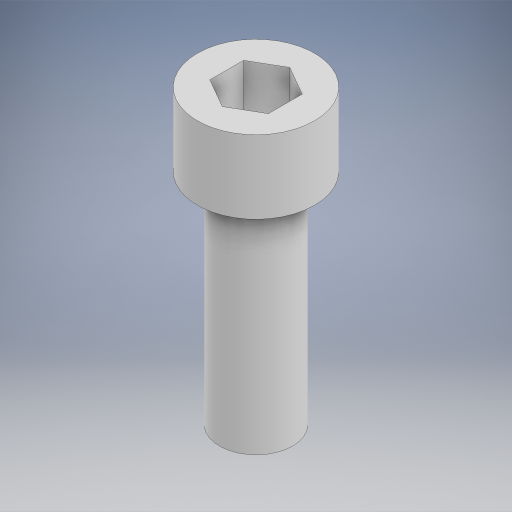
# Autodesk Inventor part: CE-2.1.5-01
Saved by Autodesk Inventor 2024 (Build 280153000, 153)
## iProperties
Created: 2024-01-31
Part Number: CE-2.1.5-01
Material: Generic
Document SubType Name: Modeling
Designer: Alex
Density: 1 g/cm^3
Appearance: Default
Author: Alex
Autodesk Inventor part; units mm, degrees
ref_plane "YZ Plane" through (0, 0, 0) normal (1, 0, 0) x (0, 1, 0)
ref_plane "XZ Plane" through (0, 0, 0) normal (0, 1, 0) x (-1, 0, 0)
ref_plane "XY Plane" through (0, 0, 0) normal (0, 0, 1) x (1, 0, 0)
sketch "Sketch1" plane through (0, 0, 0) normal (0, 0, 1) x (1, 0, 0)
  line L0 (0, 0) -> (0, 80)
  line L1 (0, 80) -> (16, 80)
  line L2 (16, 80) -> (16, 60)
  line L3 (16, 60) -> (10, 60)
  line L4 (10, 60) -> (10, 0)
  line L5 (0, 0) -> (10, 0)
  dimension "d" = 20
  dimension "HT" = 20
  dimension "Height" = 60
  dimension "HD" = 32
  constraints: 12 end point, 4 perpendicular, 1 horizontal, 1 vertical
  measures "d" diameter of L4 L0
  measures "HT" distance of L1.end L2.end
  measures "Height" distance of L3.end L4.end
  measures "HD" diameter of L2 L0
revolve "Revolution1" add sketch "Sketch1" angle 360 about axis through (0, 0, 0) along (0, 1, 0)
sketch "Sketch2" plane through (0, 80, 0) normal (0, 1, 0) x (1, 0, 0)
  line L0 (0, 9.2376) -> (8, 4.6188)
  line L1 (8, 4.6188) -> (8, -4.6188)
  line L2 (8, -4.6188) -> (0, -9.2376)
  line L3 (0, -9.2376) -> (-8, -4.6188)
  line L4 (-8, -4.6188) -> (-8, 4.6188)
  line L5 (-8, 4.6188) -> (0, 9.2376)
  point P0 (0, 0)
  point P1 (0, 0)
  dimension "HL" = 16
  constraints: 12 end point, 1 coincident, 1 vertical, 13 other
  measures "HL" distance between parallel lines of L1 L4
extrude "Extrusion1" cut sketch "Sketch2" against normal blind 12
equation "\"HT\" = d"
equation "\"Height\" = 3 * d"
equation "\"HD\" = 1.6 * d"
equation "\"HL\" = 0.8 * d"
equation "\"HH\" = 0.6 * d"
body "Solid1"
